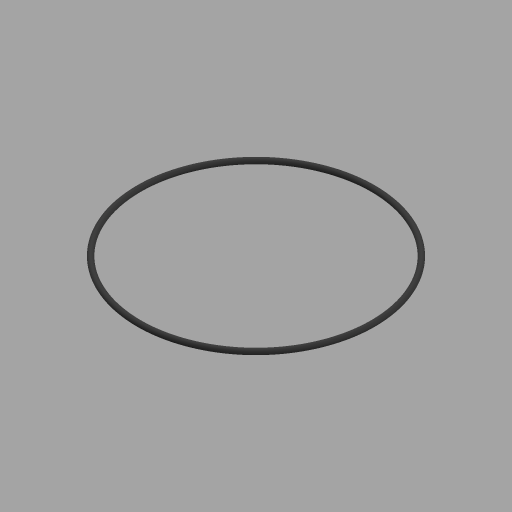
# Autodesk Inventor part: RubberOringD3.5XD156
Saved by Autodesk Inventor 2024 (Build 280153020, 153B)
## iProperties
Created: 2023-10-25
Part Number: RubberOringD3.5XD156
Material: Rubber
Document SubType Name: Modeling
Designer: schanen
Density: 0.93 g/cm^3
Appearance: Rubber - Black
Author: schanen
Autodesk Inventor part; units mm, degrees
ref_plane "YZ Plane" through (0, 0, 0) normal (1, 0, 0) x (0, 1, 0)
ref_plane "XZ Plane" through (0, 0, 0) normal (0, 1, 0) x (-1, 0, 0)
ref_plane "XY Plane" through (0, 0, 0) normal (0, 0, 1) x (1, 0, 0)
sketch "Sketch1" plane through (0, 0, 0) normal (0, 0, 1) x (1, 0, 0)
  circle A0 centre (-78, 0) radius 1.75
  line L0 (0, -2.45) -> (0, 2.45) projected
  point P0 (0, 0)
  dimension "d0" = 3.5
  dimension "d1" = 78
  constraints: 1 centre point, 1 horizontal alignment
  measures "d0" diameter of A0
  measures "d1" distance of point (0, 0) A0.centre
revolve "Revolution1" add sketch "Sketch1" angle 360 about axis through (0, -10, 0) along (0, 1, 0)
body "Solid1"
